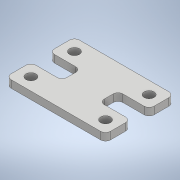
# Autodesk Inventor part: mountT
Saved by Autodesk Inventor 2021.1 (Build 251245010, 245A)
## iProperties
Created: 2017-12-07
Part Number: mountT
Material: 一般
Document SubType Name: Modeling
Designer: gisen
Density: 1 g/cm^3
Appearance: 既定
Author: gisen
Autodesk Inventor part; units mm, degrees
ref_plane "YZ Plane" through (0, 0, 0) normal (1, 0, 0) x (0, 1, 0)
ref_plane "XZ Plane" through (0, 0, 0) normal (0, 1, 0) x (-1, 0, 0)
ref_plane "XY Plane" through (0, 0, 0) normal (0, 0, 1) x (1, 0, 0)
sketch "スケッチ1" plane through (0, 0, 0) normal (0, 0, 1) x (1, 0, 0)
  line L0 (0, 0) -> (40, 0)
  line L1 (40, 0) -> (40, 10)
  line L2 (40, 10) -> (0, 10)
  line L3 (0, 10) -> (0, 0)
  line L4 (12.5, 17.5) -> (27.5, 17.5)
  line L5 (27.5, 17.5) -> (27.5, 10)
  line L6 (27.5, 10) -> (12.5, 10)
  line L7 (12.5, 10) -> (12.5, 17.5)
  line L8 (0, 17.5) -> (40, 17.5)
  line L9 (40, 17.5) -> (40, 27.5)
  line L10 (40, 27.5) -> (0, 27.5)
  line L11 (0, 27.5) -> (0, 17.5)
  circle A0 centre (5, 5) radius 2
  circle A1 centre (35, 5) radius 2
  circle A2 centre (5, 22.5) radius 2
  circle A3 centre (35, 22.5) radius 2
  point P0 (40, 22.5)
  point P1 (0, 5)
  point P2 (40, 5)
  point P3 (20, 17.5)
  point P4 (12.5, 20)
  point P5 (27.5, 20)
  dimension "d0" = 40
  dimension "d1" = 10
  dimension "d2" = 7.5
  dimension "d3" = 15
  dimension "d4" = 12.5
  dimension "d5" = 40
  dimension "d6" = 10
  dimension "d8" = 12.5
  dimension "d9" = 4
  dimension "d10" = 4
  dimension "d11" = 4
  dimension "d12" = 4
  dimension "d16" = 5
  dimension "d17" = 5
  dimension "d25" = 7.5
  constraints: 24 end point, 6 parallel, 4 centre point, 4 horizontal alignment, 4 midpoint, 3 horizontal, 3 perpendicular, 3 point on line, 2 vertical alignment
  measures "d0" distance of L2.end L1.end
  measures "d1" distance of L1.end L0.end
  measures "d2" distance of L4.end L5.end
  measures "d3" distance between parallel lines of L7 L5
  measures "d4" distance between parallel lines of L3 L7
  measures "d5" distance of L10.end L9.end
  measures "d6" distance of L9.end L8.end
  measures "d8" distance between parallel lines of L7 L11
  measures "d9" diameter of A0
  measures "d10" diameter of A1
  measures "d11" diameter of A2
  measures "d12" diameter of A3
  measures "d16" distance from line of L11 A2.centre
  measures "d17" distance from line of L9 A3.centre
  measures "d25" distance between parallel lines of L8 L6
extrude "押し出し1" add sketch "スケッチ1" along normal blind 3
fillet "フィレット1" radius 2 12 edges at (40, 27.5, 1.5) (40, 17.5, 1.5) (0, 27.5, 1.5) (0, 17.5, 1.5) (12.5, 17.5, 1.5) (27.5, 17.5, 1.5) (27.5, 10, 1.5) (40, 10, 1.5) (40, 0, 1.5) (12.5, 10, 1.5) (0, 10, 1.5) (0, 0, 1.5)
equation "\"d8\" = d4"
